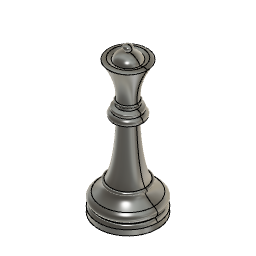
Queen Chess Piece v1 (Autodesk Fusion 360 design; units mm, degrees)
Autodesk Fusion 360 part; units mm, degrees
sketch "Sketch1" plane through (0, 0, 0) normal (0, 1, 0) x (1, 0, 0)
  spline S0 degree 5 poles (0, -59.6771) (0.0625, -59.6725) (0.1853, -59.6616) (0.3625, -59.6397) (0.5849, -59.5996) (0.8385, -59.5309) (1.0658, -59.4426) (1.2637, -59.3338) (1.4275, -59.2036) (1.5513, -59.0513) (1.6287, -58.8762) (1.6533, -58.6782) (1.6203, -58.4573) (1.5274, -58.2138) (1.3749, -57.9488) (1.1639, -57.6632) (0.9497, -57.4188) (0.7642, -57.2269) (0.6295, -57.0951) (0.5594, -57.0282) knots 0 0 0 0 0 0 0.066667 0.133333 0.2 0.266667 0.333333 0.4 0.466667 0.533333 0.6 0.666667 0.733333 0.8 0.866667 0.933333 1 1 1 1 1 1
  spline S1 degree 5 poles (4.8974, -54.3409) (4.8695, -54.4185) (4.8096, -54.5714) (4.7079, -54.7942) (4.5483, -55.0781) (4.3084, -55.4101) (4.0282, -55.7182) (3.7096, -56.0006) (3.3572, -56.2554) (2.9799, -56.4807) (2.5903, -56.6745) (2.203, -56.8348) (1.8323, -56.9599) (1.4913, -57.0484) (1.1894, -57.0997) (0.9309, -57.1143) (0.76, -57.0973) (0.6519, -57.0688) (0.5887, -57.0429) (0.5594, -57.0282) knots 0 0 0 0 0 0 0.066667 0.133333 0.2 0.266667 0.333333 0.4 0.466667 0.533333 0.6 0.666667 0.733333 0.8 0.866667 0.933333 1 1 1 1 1 1
  spline S2 degree 5 poles (4.8974, -54.3409) (4.9542, -54.3609) (5.0679, -54.4008) (5.2383, -54.4607) (5.4656, -54.5406) (5.7497, -54.6404) (5.977, -54.7202) (6.1474, -54.7801) (6.261, -54.82) (6.3179, -54.84) knots 0 0 0 0 0 0 0.2 0.4 0.6 0.8 1 1 1 1 1 1
  spline S3 degree 5 poles (6.3179, -54.84) (6.3764, -54.8333) (6.4912, -54.8194) (6.6565, -54.7975) (6.863, -54.766) (7.096, -54.7226) (7.3014, -54.6746) (7.4763, -54.6216) (7.6184, -54.5632) (7.7272, -54.4994) (7.8045, -54.4304) (7.843, -54.3714) (7.8594, -54.3251) (7.8649, -54.2933) (7.8663, -54.2772) knots 0 0 0 0 0 0 0.1 0.2 0.3 0.4 0.5 0.6 0.7 0.8 0.9 1 1 1 1 1 1
  spline S4 degree 5 poles (7.8663, -54.2772) (7.6861, -53.9704) (7.3341, -53.3593) (6.8306, -52.4496) (6.2094, -51.2511) (5.5225, -49.7787) (4.934, -48.3346) (4.4534, -46.9215) (4.0885, -45.5416) (3.8387, -44.1948) (3.697, -42.879) (3.6639, -41.8494) (3.6815, -41.0894) (3.7117, -40.5881) (3.7315, -40.3388) knots 0 0 0 0 0 0 0.1 0.2 0.3 0.4 0.5 0.6 0.7 0.8 0.9 1 1 1 1 1 1
  spline S5 degree 5 poles (3.7315, -40.3388) (3.7586, -40.3326) (3.8111, -40.3197) (3.8849, -40.2988) (3.973, -40.2678) (4.0657, -40.2237) (4.1402, -40.1741) (4.1961, -40.1193) (4.233, -40.0598) (4.2508, -39.9966) (4.2503, -39.931) (4.2322, -39.8645) (4.1972, -39.7984) (4.1464, -39.7338) (4.0806, -39.6714) (4.0008, -39.6115) (3.9262, -39.5656) (3.8644, -39.5324) (3.8207, -39.5107) (3.7981, -39.5) knots 0 0 0 0 0 0 0.066667 0.133333 0.2 0.266667 0.333333 0.4 0.466667 0.533333 0.6 0.666667 0.733333 0.8 0.866667 0.933333 1 1 1 1 1 1
  line L0 (3.7981, -39.5) -> (3.7981, -38.4714)
  spline S6 degree 5 poles (3.7981, -38.4714) (3.8388, -38.4476) (3.9194, -38.4011) (4.0383, -38.3349) (4.1929, -38.2536) (4.379, -38.1637) (4.557, -38.0846) (4.725, -38.0144) (4.8798, -37.9493) (5.0172, -37.8829) (5.132, -37.8072) (5.2189, -37.7136) (5.2734, -37.5947) (5.2924, -37.4449) (5.275, -37.2617) (5.2214, -37.0443) (5.1501, -36.8433) (5.0811, -36.6774) (5.0282, -36.5602) (5, -36.5) knots 0 0 0 0 0 0 0.066667 0.133333 0.2 0.266667 0.333333 0.4 0.466667 0.533333 0.6 0.666667 0.733333 0.8 0.866667 0.933333 1 1 1 1 1 1
  spline S7 degree 5 poles (5, -36.5) (5.0687, -36.4654) (5.2015, -36.3954) (5.3877, -36.2885) (5.6089, -36.1417) (5.8375, -35.9507) (6.0136, -35.7516) (6.1326, -35.5437) (6.1913, -35.3263) (6.191, -35.0998) (6.136, -34.8648) (6.0514, -34.6705) (5.9667, -34.5215) (5.9008, -34.4207) (5.8656, -34.3699) knots 0 0 0 0 0 0 0.1 0.2 0.3 0.4 0.5 0.6 0.7 0.8 0.9 1 1 1 1 1 1
  spline S8 degree 5 poles (5.8656, -34.3699) (5.8086, -34.3493) (5.6954, -34.3092) (5.5281, -34.2524) (5.3101, -34.1836) (5.0467, -34.11) (4.7931, -34.0497) (4.5502, -34.0042) (4.3189, -33.9743) (4.0987, -33.9596) (3.8889, -33.9592) (3.7288, -33.9694) (3.6129, -33.9826) (3.5373, -33.9938) (3.5, -34) knots 0 0 0 0 0 0 0.1 0.2 0.3 0.4 0.5 0.6 0.7 0.8 0.9 1 1 1 1 1 1
  spline S9 degree 5 poles (3.5, -34) (3.5156, -33.5497) (3.5488, -32.6572) (3.6051, -31.3432) (3.6932, -29.6409) (3.8255, -27.5987) (3.9809, -25.6468) (4.16, -23.7914) (4.3633, -22.0401) (4.5907, -20.4008) (4.8411, -18.8811) (5.1118, -17.4874) (5.3996, -16.2251) (5.7013, -15.0986) (6.0137, -14.1106) (6.3347, -13.2612) (6.5974, -12.6903) (6.7975, -12.3221) (6.9323, -12.103) (7, -12) knots 0 0 0 0 0 0 0.066667 0.133333 0.2 0.266667 0.333333 0.4 0.466667 0.533333 0.6 0.666667 0.733333 0.8 0.866667 0.933333 1 1 1 1 1 1
  spline S10 degree 5 poles (7, -12) (7.0392, -12.0018) (7.1157, -12.003) (7.2244, -11.9978) (7.3574, -11.9766) (7.5028, -11.9262) (7.6262, -11.8519) (7.7257, -11.7552) (7.799, -11.6392) (7.8434, -11.5097) (7.856, -11.3738) (7.8341, -11.2391) (7.7754, -11.1126) (7.6789, -10.9993) (7.5449, -10.9022) (7.3744, -10.8225) (7.2096, -10.773) (7.0705, -10.7437) (6.9709, -10.7277) (6.9194, -10.7206) knots 0 0 0 0 0 0 0.066667 0.133333 0.2 0.266667 0.333333 0.4 0.466667 0.533333 0.6 0.666667 0.733333 0.8 0.866667 0.933333 1 1 1 1 1 1
  spline S11 degree 5 poles (6.9194, -10.7206) (6.9272, -10.6614) (6.9492, -10.542) (7.0013, -10.3602) (7.1093, -10.1122) (7.3127, -9.7925) (7.589, -9.4623) (7.9416, -9.1211) (8.3681, -8.7694) (8.8623, -8.408) (9.4174, -8.0378) (9.9054, -7.7353) (10.2945, -7.5052) (10.564, -7.3503) (10.7012, -7.2725) knots 0 0 0 0 0 0 0.1 0.2 0.3 0.4 0.5 0.6 0.7 0.8 0.9 1 1 1 1 1 1
  spline S12 degree 5 poles (10.7012, -7.2725) (10.7683, -7.233) (10.8991, -7.1541) (11.0854, -7.036) (11.3139, -6.879) (11.5652, -6.6834) (11.7807, -6.4881) (11.9586, -6.2927) (12.0972, -6.0961) (12.1951, -5.8968) (12.2514, -5.6927) (12.2658, -5.4818) (12.2382, -5.262) (12.1693, -5.0319) (12.0604, -4.791) (11.9131, -4.539) (11.7658, -4.3287) (11.6391, -4.1662) (11.5476, -4.0558) (11.5, -4) knots 0 0 0 0 0 0 0.066667 0.133333 0.2 0.266667 0.333333 0.4 0.466667 0.533333 0.6 0.666667 0.733333 0.8 0.866667 0.933333 1 1 1 1 1 1
  spline S13 degree 5 poles (11.5, -4) (11.4774, -3.9743) (11.4321, -3.923) (11.3642, -3.846) (11.2736, -3.7434) (11.1605, -3.6151) (11.0699, -3.5125) (11.002, -3.4355) (10.9567, -3.3842) (10.9341, -3.3585) knots 0 0 0 0 0 0 0.2 0.4 0.6 0.8 1 1 1 1 1 1
  spline S14 degree 5 poles (10.9341, -3.3585) (10.9655, -3.3661) (11.0277, -3.3783) (11.119, -3.3883) (11.2369, -3.3846) (11.3773, -3.3495) (11.5101, -3.2816) (11.6349, -3.1787) (11.7516, -3.0404) (11.8607, -2.8688) (11.9627, -2.6668) (12.0393, -2.483) (12.094, -2.3335) (12.1294, -2.2288) (12.1467, -2.1751) knots 0 0 0 0 0 0 0.1 0.2 0.3 0.4 0.5 0.6 0.7 0.8 0.9 1 1 1 1 1 1
  line L1 (12.1467, -2.1751) -> (12.1467, 0)
  line L2 (12.1467, 0) -> (0, 0)
  line L3 (0, 0) -> (0, -59.6771)
  point P0 (1.2504, -59.3316)
  point P1 (1.6343, -58.6022)
  point P2 (3.5538, -56.1069)
  point P3 (1.5495, -57.0282)
  point P4 (7.5463, -54.5905)
  point P5 (4.3317, -46.4076)
  point P6 (4.199, -40.1084)
  point P7 (4.199, -39.8077)
  point P8 (4.7502, -38.0036)
  point P9 (5.2514, -37.6278)
  point P10 (6.1323, -35.5036)
  point P11 (4.5, -34)
  point P12 (4.544, -20.7845)
  point P13 (5.8989, -14.4959)
  point P14 (7.7169, -11.7532)
  point P15 (7.7887, -11.1545)
  point P16 (7.6988, -9.3654)
  point P17 (12.0031, -6.2219)
  point P18 (12.2346, -5.2926)
  point P19 (11.596, -3.2048)
  constraint coincident L2.end L3.start
  constraint vertical L0
  constraint vertical L1
  constraint perpendicular L1 L2
  constraint perpendicular L2 L3
revolve "Revolve1" add sketch "Sketch1" angle 360 about axis through (0, 0, 0) along (0, 0, 1)
